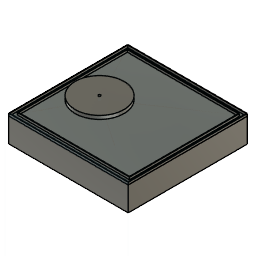
popup (Autodesk Fusion 360 design; units mm, degrees)
part number: 2026-05-09-16-28-02-982
part number: 2026-05-13-14-31-51-283
Autodesk Fusion 360 part; units mm, degrees
sketch "Sketch5" plane through (0, 0, 0) normal (0, 0, 1) x (1, 0, 0)
  line L0 (-100, 100) -> (100, 100)
  line L1 (100, 100) -> (100, -100)
  line L2 (100, -100) -> (-100, -100)
  line L3 (-100, -100) -> (-100, 100)
  constraint horizontal L0
  constraint vertical L1
  constraint horizontal L2
  constraint vertical L3
extrude "Extrude4" add sketch "Sketch5" along normal blind 2 makes body 1
sketch "Sketch8" plane through (0, 0, 2) normal (0, 0, 1) x (-1, 0, 0)
  line L0 (100, 100) -> (-100, 100)
  line L1 (-100, 100) -> (-100, -100)
  line L2 (-100, -100) -> (100, -100)
  line L3 (100, -100) -> (100, 100)
  circle A0 centre (49.4209, 0) radius 42.2465
extrude "Extrude7" add sketch "Sketch8" along normal blind 1 contours A0 bodies 1
hole "Hole2" at (-49.4209, 0, 3) direction (0, 0, -1) diameter 4 depth 35 tip angle 118 bodies 1
split "Split1" by plane through (0, 0, 2) normal (0, 0, 1) bodies 1 makes body 2 at (-78.0927, 2.1487, 3)
sketch "Sketch9" plane through (0, -100, 0) normal (0, -1, 0) x (1, 0, 0)
  line L0 (-100, 0) -> (100, 0)
  line L1 (100, 0) -> (100, 2)
  line L2 (100, 2) -> (-100, 2)
  line L3 (-100, 2) -> (-100, 0)
  line L4 (-100, 2) -> (100, 2)
  line L5 (100, 2) -> (100, -40)
  line L6 (100, -40) -> (-100, -40)
  line L7 (-100, -40) -> (-100, 2)
  constraint horizontal L4
  constraint vertical L5
  constraint horizontal L6
  constraint vertical L7
  constraint coincident L2.end L3.start
extrude "Extrude8" add sketch "Sketch9" along normal blind 3 separate body contours L0 L5 L6 L7 makes body 3
extrude "Extrude9" add 1 faces at (33.3333, -100, 1.3333) along direction (0, -1, 0) blind 3 on bodies 1 bodies 1 3
sketch "Sketch10" plane through (-100, 0, 0) normal (-1, 0, 0) x (0, -1, 0)
  line L0 (-100, 0) -> (100, 0)
  line L1 (100, 0) -> (100, -40)
  line L2 (100, -40) -> (103, -40)
  line L3 (103, -40) -> (103, 2)
  line L4 (103, 2) -> (-100, 2)
  line L5 (-100, 2) -> (-100, 0)
  line L6 (-100, 2) -> (102.906, 2)
  line L7 (102.906, 2) -> (102.906, -39.9635)
  line L8 (102.906, -39.9635) -> (-100, -39.9635)
  line L9 (-100, -39.9635) -> (-100, 2)
  constraint horizontal L6
  constraint vertical L7
  constraint horizontal L8
  constraint vertical L9
  constraint coincident L4.end L5.start
extrude "Extrude10" add sketch "Sketch10" along normal blind 3 separate body contours L0 L1 L8 L9 makes body 4
extrude "Extrude11" add 1 faces at (-100, -102, -12.6667) along direction (-1, 0, 0) blind 3 on bodies 1 bodies 1 4
sketch "Sketch11" plane through (0, 100, 0) normal (0, 1, 0) x (-1, 0, 0)
  line L0 (-100, 0) -> (100, 0)
  line L1 (100, 0) -> (100, -39.9635)
  line L2 (100, -39.9635) -> (103, -39.9635)
  line L3 (103, -39.9635) -> (103, 2)
  line L4 (103, 2) -> (-100, 2)
  line L5 (-100, 2) -> (-100, 0)
  line L6 (-100, 2) -> (103, 2)
  line L7 (103, 2) -> (103, -39.9635)
  line L8 (103, -39.9635) -> (-100, -39.9635)
  line L9 (-100, -39.9635) -> (-100, 2)
  constraint horizontal L6
  constraint vertical L7
  constraint horizontal L8
  constraint vertical L9
  constraint coincident L2.end L3.start
  constraint coincident L4.end L5.start
extrude "Extrude13" add 1 faces at (-102, 100, -12.6545) along direction (0, 1, 0) blind 3 on bodies 1 bodies 1
sketch "Sketch12" plane through (0, 0, 2) normal (0, 0, 1) x (-1, 0, 0)
  circle A0 centre (49.4209, 0) radius 2
  line L0 (-100, 103) -> (-100, -103)
  line L1 (-100, -103) -> (103, -103)
  line L2 (103, -103) -> (103, 103)
  line L3 (103, 103) -> (-100, 103)
sketch "Sketch13" plane through (100, 0, 0) normal (1, 0, 0) x (0, 1, 0)
  line L0 (-100, 0) -> (103, 0)
  line L1 (103, 0) -> (103, 2)
  line L2 (103, 2) -> (-103, 2)
  line L3 (-103, 2) -> (-103, -40)
  line L4 (-103, -40) -> (-100, -40)
  line L5 (-100, -40) -> (-100, 0)
  line L6 (-103, 2) -> (102.8044, 2)
  line L7 (102.8044, 2) -> (102.8044, -39.9323)
  line L8 (102.8044, -39.9323) -> (-103, -39.9323)
  line L9 (-103, -39.9323) -> (-103, 2)
  constraint horizontal L6
  constraint vertical L7
  constraint horizontal L8
  constraint vertical L9
  constraint coincident L2.end L3.start
extrude "Extrude14" add sketch "Sketch13" along normal blind 3 separate body contours L0 L5 L7 L8 makes body 5
extrude "Extrude15" add 1 faces at (100, -102, -12.6667) along direction (1, 0, 0) blind 3 on bodies 1 bodies 1 5
sketch "Sketch14" plane through (0, 0, 2) normal (0, 0, 1) x (1, 0, 0)
  line L0 (102.9396, -102.7347) -> (-103.1444, -102.7347)
  line L1 (-103.1444, -102.7347) -> (-103.1444, 102.5299)
  line L2 (-103.1444, 102.5299) -> (102.9396, 102.5299)
  line L3 (102.9396, 102.5299) -> (102.9396, -102.7347)
  line L4 (-96.7313, -93.9576) -> (-96.7313, 95.4105)
  line L5 (-96.7313, 95.4105) -> (96.2885, 95.4105)
  line L6 (96.2885, 95.4105) -> (96.2885, -93.9576)
  line L7 (96.2885, -93.9576) -> (-96.7313, -93.9576)
  constraint horizontal L0
  constraint vertical L1
  constraint horizontal L2
  constraint vertical L3
  constraint perpendicular L4 L5
  constraint parallel L4 L6
  constraint parallel L5 L7
  constraint perpendicular L2 L4
extrude "Extrude1" add sketch "Sketch14" along normal mid plane 4 from surface at 2 thin wall 1 centred separate body makes body 6 at (-34.6164, -103.2347, 4.6667) makes body 7 at (-32.558, -94.4576, 4.6667) in component "Component"
extrude "Extrude16" add 1 faces at (-103, -33.3333, -11.9878) along direction (-1, 0, 0) blind 1 on bodies 1 bodies 1
extrude "Extrude17" cut 1 faces at (-104, -33.3333, -11.9878) along direction (1, 0, 0) blind 0.5 on bodies 1 bodies 1
extrude "Extrude18" add 1 faces at (-103.5, -33.3333, -11.9878) along direction (-1, 0, 0) blind 0.155 on bodies 1 bodies 1
extrude "Extrude19" add 1 faces at (34.115, -103, -12) along direction (0, -1, 0) blind 0.235 on bodies 1 bodies 1
extrude "Extrude20" add 1 faces at (103, -33.4769, -12.6441) along direction (1, 0, 0) blind 0.44 on bodies 1 bodies 1
extrude "Extrude21" cut 1 faces at (-103.655, -33.4117, -11.9878) along direction (1, 0, 0) blind 0.011 on bodies 1 bodies 1
extrude "Extrude22" add 1 faces at (-78.0927, 2.1487, 3) along direction (0, 0, 1) blind 5 on bodies 2 bodies 2
sketch "Sketch15" plane through (0, -102.2347, 0) normal (0, 1, 0) x (-1, 0, 0)
  line L0 (102.6444, 2) -> (102.6444, 6)
  line L1 (102.6444, 6) -> (-102.4396, 6)
  line L2 (-102.4396, 6) -> (-102.4396, 2)
  line L3 (-102.4396, 2) -> (102.6444, 2)
sketch "Sketch16" plane through (0, 0, 2) normal (0, 0, 1) x (-1, 0, 0)
sketch "Sketch17" plane through (0, 0, 2) normal (0, 0, 1) x (-1, 0, 0)
sketch "Sketch18" plane through (0, 0, 0) normal (0, 1, 0) x (1, 0, 0)
component "Component" placed x (1, 0, 0) y (0, 1, 0) z (0, 0, 1) at (0, 0, 0)
named bodies: "base", "base (1)"
